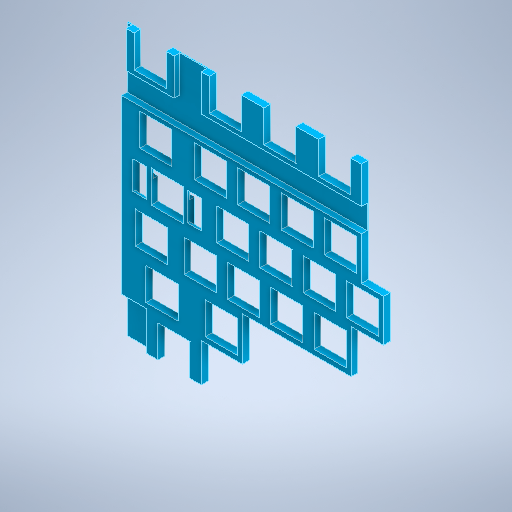
# Autodesk Inventor part: Upper Left Plate
Saved by Autodesk Inventor 2025 (Build 290162000, 162)
## iProperties
Created: 2024-06-29
Part Number: Upper Left Plate
Material: PET Plastic
Document SubType Name: Modeling
Designer: adam
Density: 1.541 g/cm^3
Appearance: Sky Blue Medium
Author: adam
Autodesk Inventor part; units mm, degrees
ref_plane "YZ Plane" through (0, 0, 0) normal (1, 0, 0) x (0, 1, 0)
ref_plane "XZ Plane" through (0, 0, 0) normal (0, 1, 0) x (-1, 0, 0)
ref_plane "XY Plane" through (0, 0, 0) normal (0, 0, 1) x (1, 0, 0)
sketch "Sketch1" plane through (0, 0, 0) normal (0, 0, 1) x (1, 0, 0)
  line L0 (157.5, 62.5) -> (-157.5, 62.5) construction
  line L1 (-157.5, 62.5) -> (-157.5, -62.5) construction
  line L2 (-157.5, -62.5) -> (157.5, -62.5) construction
  line L3 (-52.25, 62.5) -> (-52.25, 14.2)
  line L4 (-52.25, 14.2) -> (-42.5, 14.2)
  line L5 (-42.5, 14.2) -> (-42.5, -4.4)
  line L6 (-42.5, -4.4) -> (-56.75, -4.4)
  line L7 (-56.75, -4.4) -> (-56.75, -23.5)
  line L8 (-56.75, -23.5) -> (-104.5, -23.5)
  line L9 (-104.5, -23.5) -> (-104.5, -42.6375)
  line L10 (-104.5, -42.6375) -> (-122.5, -42.6375)
  line L11 (-122.5, -42.6375) -> (-122.5, -62.5)
  line L12 (-122.5, -62.5) -> (-157.5, -62.5)
  line L13 (-157.5, -62.5) -> (-157.5, 62.5)
  line L14 (-157.5, 62.5) -> (-52.25, 62.5)
  line L15 (-51.75, 61.525) -> (-51.75, 43.475) construction
  line L16 (-51.75, 14.7) -> (-42, 14.7) construction
  line L17 (-42, 14.7) -> (-42, -4.9) construction
  line L18 (-42, -4.9) -> (-56.25, -4.9) construction
  line L19 (-56.25, -4.9) -> (-56.25, -23.5) construction
  line L20 (66.5, -24) -> (-104, -24) construction
  line L21 (-104, -24) -> (-104, -43.1375) construction
  line L22 (-104, -43.1375) -> (-122, -43.1375) construction
  line L23 (-122, -43.1375) -> (-122, -62.5) construction
  line L24 (-152.025, 45.475) -> (-152.025, 59.525) projected
  line L25 (-152.025, 59.525) -> (-137.975, 59.525) projected
  line L26 (-137.975, 59.525) -> (-137.975, 45.475) projected
  line L27 (-137.975, 45.475) -> (-152.025, 45.475) projected
  line L28 (-119.025, 45.475) -> (-119.025, 59.525) projected
  line L29 (-119.025, 59.525) -> (-104.975, 59.525) projected
  line L30 (-104.975, 59.525) -> (-104.975, 45.475) projected
  line L31 (-104.975, 45.475) -> (-119.025, 45.475) projected
  line L32 (-95.025, 45.475) -> (-95.025, 59.525) projected
  line L33 (-95.025, 59.525) -> (-80.975, 59.525) projected
  line L34 (-80.975, 59.525) -> (-80.975, 45.475) projected
  line L35 (-80.975, 45.475) -> (-95.025, 45.475) projected
  line L36 (-71.025, 59.525) -> (-56.975, 59.525) projected
  line L37 (-56.975, 59.525) -> (-56.975, 45.475) projected
  line L38 (-56.975, 45.475) -> (-71.025, 45.475) projected
  line L39 (-71.025, 45.475) -> (-71.025, 59.525) projected
  line L40 (-68.525, 31.025) -> (-54.475, 31.025) projected
  line L41 (-54.475, 31.025) -> (-54.475, 16.975) projected
  line L42 (-68.525, 16.975) -> (-68.525, 31.025) projected
  line L43 (-54.475, 16.975) -> (-68.525, 16.975) projected
  line L44 (-73.475, 31.025) -> (-73.475, 16.975) projected
  line L45 (-87.525, 31.025) -> (-73.475, 31.025) projected
  line L46 (-87.525, 16.975) -> (-87.525, 31.025) projected
  line L47 (-73.475, 16.975) -> (-87.525, 16.975) projected
  line L48 (-92.475, 31.025) -> (-92.475, 16.975) projected
  line L49 (-106.525, 31.025) -> (-92.475, 31.025) projected
  line L50 (-106.525, 16.975) -> (-106.525, 31.025) projected
  line L51 (-92.475, 16.975) -> (-106.525, 16.975) projected
  line L52 (-111.475, 31.025) -> (-111.475, 16.975) projected
  line L53 (-125.525, 16.975) -> (-125.525, 31.025) projected
  line L54 (-125.525, 31.025) -> (-111.475, 31.025) projected
  line L55 (-111.475, 16.975) -> (-125.525, 16.975) projected
  line L56 (-149.525, 31.025) -> (-135.475, 31.025) projected
  line L57 (-135.475, 31.025) -> (-135.475, 16.975) projected
  line L58 (-149.525, 16.975) -> (-149.525, 31.025) projected
  line L59 (-135.475, 16.975) -> (-149.525, 16.975) projected
  line L60 (-144.525, 11.925) -> (-130.475, 11.925) projected
  line L61 (-130.475, -2.125) -> (-144.525, -2.125) projected
  line L62 (-130.475, 11.925) -> (-130.475, -2.125) projected
  line L63 (-144.525, -2.125) -> (-144.525, 11.925) projected
  line L64 (-115.775, -2.125) -> (-115.775, 11.925) projected
  line L65 (-115.775, 11.925) -> (-101.725, 11.925) projected
  line L66 (-101.725, 11.925) -> (-101.725, -2.125) projected
  line L67 (-101.725, -2.125) -> (-115.775, -2.125) projected
  line L68 (-96.775, 11.925) -> (-82.725, 11.925) projected
  line L69 (-82.725, 11.925) -> (-82.725, -2.125) projected
  line L70 (-96.775, -2.125) -> (-96.775, 11.925) projected
  line L71 (-82.725, -2.125) -> (-96.775, -2.125) projected
  line L72 (-77.775, 11.925) -> (-63.725, 11.925) projected
  line L73 (-63.725, 11.925) -> (-63.725, -2.125) projected
  line L74 (-63.725, -2.125) -> (-77.775, -2.125) projected
  line L75 (-77.775, -2.125) -> (-77.775, 11.925) projected
  line L76 (-58.775, 11.925) -> (-44.725, 11.925) projected
  line L77 (-44.725, 11.925) -> (-44.725, -2.125) projected
  line L78 (-44.725, -2.125) -> (-58.775, -2.125) projected
  line L79 (-58.775, -2.125) -> (-58.775, 11.925) projected
  line L80 (-73.025, -7.175) -> (-58.975, -7.175) projected
  line L81 (-58.975, -7.175) -> (-58.975, -21.225) projected
  line L82 (-58.975, -21.225) -> (-73.025, -21.225) projected
  line L83 (-73.025, -21.225) -> (-73.025, -7.175) projected
  line L84 (-77.975, -7.175) -> (-77.975, -21.225) projected
  line L85 (-92.025, -7.175) -> (-77.975, -7.175) projected
  line L86 (-92.025, -21.225) -> (-92.025, -7.175) projected
  line L87 (-77.975, -21.225) -> (-92.025, -21.225) projected
  line L88 (-96.975, -7.175) -> (-96.975, -21.225) projected
  line L89 (-111.025, -7.175) -> (-96.975, -7.175) projected
  line L90 (-111.025, -21.225) -> (-111.025, -7.175) projected
  line L91 (-96.975, -21.225) -> (-111.025, -21.225) projected
  line L92 (-130.025, -7.175) -> (-115.975, -7.175) projected
  line L93 (-115.975, -7.175) -> (-115.975, -21.225) projected
  line L94 (-130.025, -21.225) -> (-130.025, -7.175) projected
  line L95 (-115.975, -21.225) -> (-130.025, -21.225) projected
  line L96 (-120.775, -26.275) -> (-106.725, -26.275) projected
  line L97 (-106.725, -26.275) -> (-106.725, -40.325) projected
  line L98 (-106.725, -40.325) -> (-120.775, -40.325) projected
  line L99 (-120.775, -40.325) -> (-120.775, -26.275) projected
  line L100 (-141.525, -45.45) -> (-127.475, -45.45) projected
  line L101 (-127.475, -45.45) -> (-127.475, -59.5) projected
  line L102 (-141.525, -59.5) -> (-141.525, -45.45) projected
  line L103 (-127.475, -59.5) -> (-141.525, -59.5) projected
  line L104 (-132.725, -26.275) -> (-132.725, -40.325) projected
  line L105 (-146.775, -26.275) -> (-132.725, -26.275) projected
  line L106 (-146.775, -40.325) -> (-146.775, -26.275) projected
  line L107 (-132.725, -40.325) -> (-146.775, -40.325) projected
  line L108 (-137.475, -7.175) -> (-137.475, -21.225) projected
  line L109 (-151.525, -21.225) -> (-151.525, -7.175) projected
  line L110 (-137.475, -21.225) -> (-151.525, -21.225) projected
  line L111 (-151.525, -7.175) -> (-137.475, -7.175) projected
  line L112 (-152.525, -3.625) -> (-152.525, 13.425) construction
  line L113 (-146.475, 13.425) -> (-146.475, -3.625) construction
  line L114 (-128.525, -3.625) -> (-128.525, 13.425) construction
  line L115 (-122.475, 13.425) -> (-122.475, -3.625) construction
  line L116 (-152.525, 11.425) -> (-146.475, 11.425)
  line L117 (-146.475, 11.425) -> (-146.475, -0.975)
  line L118 (-146.475, -0.975) -> (-152.525, -0.975)
  line L119 (-152.525, -0.975) -> (-152.525, 11.425)
  line L120 (-128.525, 11.425) -> (-122.475, 11.425)
  line L121 (-122.475, 11.425) -> (-122.475, -0.975)
  line L122 (-122.475, -0.975) -> (-128.525, -0.975)
  line L123 (-128.525, -0.975) -> (-128.525, 11.425)
  line L124 (-152.525, 13.425) -> (-146.475, 13.425) construction
  point P0 (0, 0)
  dimension "d0" = 0.5
  dimension "d1" = 0.5
  dimension "d2" = 0.5
  dimension "d3" = 0.5
  dimension "d4" = 0.5
  dimension "d5" = 0.5
  dimension "d6" = 0.5
  dimension "d7" = 0.5
  dimension "d8" = 0.5
  dimension "d9" = 2
  dimension "d10" = 12.4
  constraints: 40 end point, 11 perpendicular, 8 point on line, 4 parallel, 2 collinear, 2 horizontal, 1 vertical
  measures "d0" distance between parallel lines of L15 L3
  measures "d1" distance between parallel lines of L4 L16
  measures "d2" distance between parallel lines of L5 L17
  measures "d3" distance between parallel lines of L18 L6
  measures "d4" distance between parallel lines of L19 L7
  measures "d5" distance between parallel lines of L20 L8
  measures "d6" distance between parallel lines of L21 L9
  measures "d7" distance between parallel lines of L22 L10
  measures "d8" distance between parallel lines of L23 L11
  measures "d9" distance between parallel lines of L116 L124
  measures "d10" distance between parallel lines of L118 L116
extrude "Extrusion1" add sketch "Sketch1" along normal blind 0.5
sketch "Sketch2" plane through (0, 0, 0.5) normal (0, 0, 1) x (1, 0, 0)
  line L0 (-155.525, 61.525) -> (-134.475, 61.525)
  line L1 (-134.475, 61.525) -> (-134.475, 43.475)
  line L2 (-134.475, 43.475) -> (-155.525, 43.475)
  line L3 (-155.525, 43.475) -> (-155.525, 61.525)
  line L4 (-122.525, 61.525) -> (-52.25, 61.525)
  line L5 (-52.25, 61.525) -> (-52.25, 43.475)
  line L6 (-52.25, 43.475) -> (-122.525, 43.475)
  line L7 (-122.525, 43.475) -> (-122.525, 61.525)
  line L8 (-157.5, 62.5) -> (-157.5, -62.5) construction
  line L9 (-157.5, 33.025) -> (-52.25, 33.025)
  line L10 (-52.25, 14.2) -> (-52.25, 62.5) construction
  line L11 (-42.5, 14.2) -> (-52.25, 14.2) construction
  line L12 (-52.25, 14.2) -> (-52.25, 62.5) projected
  line L13 (-52.25, 33.025) -> (-52.25, 14.2)
  line L14 (-42.5, -4.4) -> (-42.5, 14.2) projected
  line L15 (-52.25, 14.2) -> (-42.5, 14.2)
  line L16 (-152.025, 59.525) -> (-137.975, 59.525) projected
  line L17 (-152.025, 45.475) -> (-152.025, 59.525) projected
  line L18 (-137.975, 59.525) -> (-137.975, 45.475) projected
  line L19 (-137.975, 45.475) -> (-152.025, 45.475) projected
  line L20 (-119.025, 45.475) -> (-119.025, 59.525) projected
  line L21 (-149.525, 31.025) -> (-135.475, 31.025) projected
  line L22 (-56.75, -4.4) -> (-42.5, -4.4) projected
  line L23 (-42.5, -4.4) -> (-56.75, -4.4)
  line L24 (-104.5, -23.5) -> (-56.75, -23.5) projected
  line L25 (-56.75, -4.4) -> (-56.75, -23.5)
  line L26 (-56.75, -23.5) -> (-104.5, -23.5)
  line L27 (-122.5, -42.6375) -> (-104.5, -42.6375) projected
  line L28 (-104.5, -23.5) -> (-104.5, -42.6375)
  line L29 (-104.5, -42.6375) -> (-122.5, -42.6375)
  line L30 (-157.5, -62.5) -> (-122.5, -62.5) construction
  line L31 (-122.5, -42.6375) -> (-122.5, -62.5)
  line L32 (-119.025, 59.525) -> (-104.975, 59.525) projected
  line L33 (-104.975, 59.525) -> (-104.975, 45.475) projected
  line L34 (-104.975, 45.475) -> (-119.025, 45.475) projected
  line L35 (-95.025, 45.475) -> (-95.025, 59.525) projected
  line L36 (-95.025, 59.525) -> (-80.975, 59.525) projected
  line L37 (-80.975, 59.525) -> (-80.975, 45.475) projected
  line L38 (-80.975, 45.475) -> (-95.025, 45.475) projected
  line L39 (-71.025, 45.475) -> (-71.025, 59.525) projected
  line L40 (-71.025, 59.525) -> (-56.975, 59.525) projected
  line L41 (-56.975, 59.525) -> (-56.975, 45.475) projected
  line L42 (-56.975, 45.475) -> (-71.025, 45.475) projected
  line L43 (-68.525, 31.025) -> (-54.475, 31.025) projected
  line L44 (-54.475, 31.025) -> (-54.475, 16.975) projected
  line L45 (-54.475, 16.975) -> (-68.525, 16.975) projected
  line L46 (-68.525, 16.975) -> (-68.525, 31.025) projected
  line L47 (-73.475, 31.025) -> (-73.475, 16.975) projected
  line L48 (-87.525, 31.025) -> (-73.475, 31.025) projected
  line L49 (-87.525, 16.975) -> (-87.525, 31.025) projected
  line L50 (-73.475, 16.975) -> (-87.525, 16.975) projected
  line L51 (-92.475, 31.025) -> (-92.475, 16.975) projected
  line L52 (-106.525, 31.025) -> (-92.475, 31.025) projected
  line L53 (-106.525, 16.975) -> (-106.525, 31.025) projected
  line L54 (-92.475, 16.975) -> (-106.525, 16.975) projected
  line L55 (-111.475, 31.025) -> (-111.475, 16.975) projected
  line L56 (-125.525, 31.025) -> (-111.475, 31.025) projected
  line L57 (-125.525, 16.975) -> (-125.525, 31.025) projected
  line L58 (-111.475, 16.975) -> (-125.525, 16.975) projected
  line L59 (-135.475, 31.025) -> (-135.475, 16.975) projected
  line L60 (-149.525, 16.975) -> (-149.525, 31.025) projected
  line L61 (-135.475, 16.975) -> (-149.525, 16.975) projected
  line L62 (-144.525, 11.925) -> (-130.475, 11.925) projected
  line L63 (-130.475, -2.125) -> (-144.525, -2.125) projected
  line L64 (-144.525, -2.125) -> (-144.525, 11.925) projected
  line L65 (-130.475, 11.925) -> (-130.475, -2.125) projected
  line L66 (-146.475, 11.425) -> (-146.475, -0.975) projected
  line L67 (-152.525, 11.425) -> (-146.475, 11.425) projected
  line L68 (-152.525, -0.975) -> (-152.525, 11.425) projected
  line L69 (-146.475, -0.975) -> (-152.525, -0.975) projected
  line L70 (-128.525, 11.425) -> (-122.475, 11.425) projected
  line L71 (-122.475, 11.425) -> (-122.475, -0.975) projected
  line L72 (-128.525, -0.975) -> (-128.525, 11.425) projected
  line L73 (-122.475, -0.975) -> (-128.525, -0.975) projected
  line L74 (-115.775, -2.125) -> (-115.775, 11.925) projected
  line L75 (-115.775, 11.925) -> (-101.725, 11.925) projected
  line L76 (-101.725, 11.925) -> (-101.725, -2.125) projected
  line L77 (-101.725, -2.125) -> (-115.775, -2.125) projected
  line L78 (-96.775, -2.125) -> (-96.775, 11.925) projected
  line L79 (-96.775, 11.925) -> (-82.725, 11.925) projected
  line L80 (-82.725, 11.925) -> (-82.725, -2.125) projected
  line L81 (-82.725, -2.125) -> (-96.775, -2.125) projected
  line L82 (-77.775, 11.925) -> (-63.725, 11.925) projected
  line L83 (-63.725, 11.925) -> (-63.725, -2.125) projected
  line L84 (-63.725, -2.125) -> (-77.775, -2.125) projected
  line L85 (-77.775, -2.125) -> (-77.775, 11.925) projected
  line L86 (-58.775, 11.925) -> (-44.725, 11.925) projected
  line L87 (-44.725, 11.925) -> (-44.725, -2.125) projected
  line L88 (-44.725, -2.125) -> (-58.775, -2.125) projected
  line L89 (-58.775, -2.125) -> (-58.775, 11.925) projected
  line L90 (-73.025, -7.175) -> (-58.975, -7.175) projected
  line L91 (-58.975, -7.175) -> (-58.975, -21.225) projected
  line L92 (-58.975, -21.225) -> (-73.025, -21.225) projected
  line L93 (-73.025, -21.225) -> (-73.025, -7.175) projected
  line L94 (-92.025, -7.175) -> (-77.975, -7.175) projected
  line L95 (-77.975, -7.175) -> (-77.975, -21.225) projected
  line L96 (-92.025, -21.225) -> (-92.025, -7.175) projected
  line L97 (-77.975, -21.225) -> (-92.025, -21.225) projected
  line L98 (-96.975, -7.175) -> (-96.975, -21.225) projected
  line L99 (-111.025, -7.175) -> (-96.975, -7.175) projected
  line L100 (-111.025, -21.225) -> (-111.025, -7.175) projected
  line L101 (-96.975, -21.225) -> (-111.025, -21.225) projected
  line L102 (-130.025, -7.175) -> (-115.975, -7.175) projected
  line L103 (-115.975, -7.175) -> (-115.975, -21.225) projected
  line L104 (-115.975, -21.225) -> (-130.025, -21.225) projected
  line L105 (-130.025, -21.225) -> (-130.025, -7.175) projected
  line L106 (-137.475, -7.175) -> (-137.475, -21.225) projected
  line L107 (-151.525, -7.175) -> (-137.475, -7.175) projected
  line L108 (-151.525, -21.225) -> (-151.525, -7.175) projected
  line L109 (-137.475, -21.225) -> (-151.525, -21.225) projected
  line L110 (-146.775, -26.275) -> (-132.725, -26.275) projected
  line L111 (-132.725, -26.275) -> (-132.725, -40.325) projected
  line L112 (-146.775, -40.325) -> (-146.775, -26.275) projected
  line L113 (-132.725, -40.325) -> (-146.775, -40.325) projected
  line L114 (-120.775, -26.275) -> (-106.725, -26.275) projected
  line L115 (-106.725, -26.275) -> (-106.725, -40.325) projected
  line L116 (-120.775, -40.325) -> (-120.775, -26.275) projected
  line L117 (-106.725, -40.325) -> (-120.775, -40.325) projected
  line L118 (-141.525, -45.45) -> (-127.475, -45.45) projected
  line L119 (-127.475, -45.45) -> (-127.475, -59.5) projected
  line L120 (-127.475, -59.5) -> (-141.525, -59.5) projected
  line L121 (-141.525, -59.5) -> (-141.525, -45.45) projected
  line L122 (-157.5, -42.5) -> (-146.5, -42.5)
  line L123 (-146.5, -42.5) -> (-146.5, -62.5)
  line L124 (-157.5, -42.5) -> (-157.5, 33.025)
  line L125 (-146.5, -62.5) -> (-122.5, -62.5)
  point P0 (0, 0)
  dimension "d13" = 2
  dimension "d14" = 3.5
  dimension "d15" = 3.5
  dimension "d16" = 2
  dimension "d17" = 3.5
  dimension "d18" = 2
  dimension "d26" = 11
  dimension "d27" = 20
  constraints: 42 end point, 7 perpendicular, 6 collinear, 5 horizontal, 5 point on line, 4 parallel
  measures "d13" distance between parallel lines of L16 L0
  measures "d14" distance between parallel lines of L17 L3
  measures "d15" distance between parallel lines of L1 L18
  measures "d16" distance between parallel lines of L19 L2
  measures "d17" distance between parallel lines of L20 L7
  measures "d18" distance between parallel lines of L9 L21
  measures "d26" distance between parallel lines of L8 L123
  measures "d27" distance between parallel lines of L30 L122
extrude "Extrusion2" add sketch "Sketch2" along normal blind 2.5
sketch "Sketch3" plane through (0, 0, 0) normal (0, 0, -1) x (-1, 0, 0)
  line L0 (122.475, -3.625) -> (122.475, 13.425) construction
  line L1 (128.525, 13.425) -> (128.525, -3.625) construction
  line L2 (146.475, -3.625) -> (146.475, 13.425) construction
  line L3 (152.525, 13.425) -> (152.525, -3.625) construction
  line L4 (122.475, -2.975) -> (128.525, -2.975)
  line L5 (128.525, -2.975) -> (128.525, 7.425)
  line L6 (128.525, 14.425) -> (122.475, 14.425)
  line L7 (122.475, 14.425) -> (122.475, -2.975)
  line L8 (146.475, 11.425) -> (146.475, -0.975) projected
  line L9 (146.475, -2.975) -> (152.525, -2.975)
  line L10 (152.525, -2.975) -> (152.525, 14.425)
  line L11 (152.525, 14.425) -> (146.475, 14.425)
  line L12 (146.475, 7.425) -> (146.475, -2.975)
  line L13 (122.475, -0.975) -> (128.525, -0.975) construction
  line L14 (128.525, 11.425) -> (122.475, 11.425) construction
  line L15 (128.525, 14.425) -> (146.475, 14.425)
  line L16 (128.525, 7.425) -> (146.475, 7.425)
  point P0 (0, 0)
  dimension "d21" = 2
  dimension "d22" = 3
  dimension "d23" = 4
  constraints: 20 end point, 5 point on line, 4 parallel, 3 horizontal, 3 perpendicular, 2 collinear
  measures "d21" distance between parallel lines of L4 L13
  measures "d22" distance between parallel lines of L14 L6
  measures "d23" distance between parallel lines of L16 L14
extrude "Extrusion3" cut sketch "Sketch3" against normal blind 2
sketch "Sketch4" plane through (0, 0, 3) normal (0, 0, 1) x (1, 0, 0)
  line L0 (-127.475, -59.5) -> (-141.525, -59.5) construction
  line L1 (-157.5, -42.5) -> (-157.5, -62.5) projected
  line L2 (-122.5, -62.5) -> (-122.5, -42.6375) projected
  line L3 (-157.5, -62.5) -> (-122.5, -62.5)
  line L4 (-122.5, -62.5) -> (-122.5, -59.5)
  line L5 (-122.5, -59.5) -> (-157.5, -59.5)
  line L6 (-157.5, -59.5) -> (-157.5, -62.5)
  line L7 (-119.025, 59.525) -> (-104.975, 59.525) projected
  line L8 (-52.25, 43.475) -> (-52.25, 61.525) projected
  line L9 (-157.5, 62.5) -> (-52.25, 62.5)
  line L10 (-52.25, 62.5) -> (-52.25, 59.525)
  line L11 (-52.25, 59.525) -> (-157.5, 59.525)
  line L12 (-157.5, 59.525) -> (-157.5, 62.5)
  point P0 (0, 0)
  constraints: 16 end point, 4 parallel, 2 collinear, 2 horizontal, 2 perpendicular, 2 point on line
extrude "Extrusion4" cut sketch "Sketch4" against normal up to surface (3 mm away)
equation "\"d0\" = dpg"
equation "\"d1\" = dpg"
equation "\"d2\" = dpg"
equation "\"d3\" = dpg"
equation "\"d4\" = dpg"
equation "\"d5\" = dpg"
equation "\"d6\" = dpg"
equation "\"d7\" = dpg"
equation "\"d8\" = dpg"
equation "\"d15\" = d14"
equation "\"d16\" = d13"
equation "\"d17\" = d14"
equation "\"d18\" = d13"
equation "\"dpg\" = 0.5"
body "Solid1"
